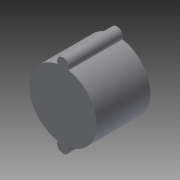
# Autodesk Inventor part: BallCaster
Saved by Autodesk Inventor 2015 (Build 190159000, 159)
## iProperties
Created: 2015-04-05
Part Number: BallCaster
Material: Generic
Document SubType Name: Modeling
Designer: Jesse
Density: 1 g/cm^3
Appearance: Default
Author: Jesse
Autodesk Inventor part; units mm, degrees
ref_plane "YZ Plane" through (0, 0, 0) normal (1, 0, 0) x (0, 1, 0)
ref_plane "XZ Plane" through (0, 0, 0) normal (0, 1, 0) x (-1, 0, 0)
ref_plane "XY Plane" through (0, 0, 0) normal (0, 0, 1) x (1, 0, 0)
sketch "Sketch1" plane through (0, 0, 0) normal (0, 1, 0) x (-1, 0, 0)
  circle A0 centre (0, 0) radius 6.35
  circle A1 centre (0, -6.731) radius 1.143
  circle A2 centre (0, 6.731) radius 1.143
  dimension "d0" = 12.7
  dimension "d1" = 2.286
  dimension "d2" = 2.286
  dimension "d3" = 6.731
  dimension "d4" = 6.731
  dimension "d5" = 13.462
  constraints: 3 centre point, 1 coincident
  measures "d0" diameter of A0
  measures "d1" diameter of A1
  measures "d2" diameter of A2
  measures "d3" distance of point (0, 0) A2.centre
  measures "d4" distance of point (0, 0) A1.centre
  measures "d5" distance of A2.centre A1.centre
extrude "Extrusion1" add sketch "Sketch1" along normal blind 10.16
body "Solid1"
